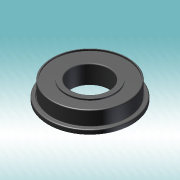
# Autodesk Inventor part: C-SFL6901ZZ
Saved by Autodesk Inventor 2015 (Build 190159000, 159)
## iProperties
Category: PARTsolutions
Company: MISUMI
Created: 2016-03-21
Part Number: C-SFL6901ZZ
Catalog Web Link: www.cadenas.de
Description: C-SFL6__ZZ, C-SFL6__AZZ, C-SFL6___ZZ-C-VALUE Stainless Steel Deep Groove Ball Bearings with Flange - Double Shielded
Vendor: MISUMI
Document SubType Name: Modeling
Designer: psAdmin
Manufacturer: MISUMI
Mass: 1.96986 g
Surface Area: 16.7276 cm^2
Volume: 1.96986 cm^3
Density: 1 g/cm^3
Material: 一般
Appearance: PSOLRGB-175-175-175
PSOL_IDENT_0: {$CADENAS_DATA\23d-libs\misumi\metric\12_bearing_holders\12_cn\c_sfl673zz.prj},195 {VTYP=3D},{NB=C-S
PSOL_IDENT_1: FL6901ZZ},{LINA=C-SFL6901ZZ},{NN=C-SFL6__ZZ, C-SFL6__AZZ, C-SFL6___ZZ},{DATE=21.07.2015 12:46:03},{G
PSOL_IDENT_2: EOMDATE=01.08.2014 01:01:00},{VERSION=},{LINEID=430},{LINESUBID=-1},{WBVAR=}  {NB=C-SFL6901ZZ},{LINA=
PSOL_IDENT_3: C-SFL6901ZZ},{KT=DUMMY},{PN=C-SFL6901ZZ},{TYPE=C-SFL6901ZZ},{BN=6901ZZ},{DD=12.0},{D=24},{B=6.0},{D1=
PSOL_IDENT_4: 26.5},{C=1.5},{RR=0.30},{B11=0.438},{D11=15.430},{D22=23.040}
NN: C-SFL6__ZZ, C-SFL6__AZZ, C-SFL6___ZZ
NT: C-VALUE Stainless Steel Deep Groove Ball Bearings with Flange - Double Shielded
NB: C-SFL6901ZZ
NBSYN: $PN.
LINA: C-SFL6901ZZ
PN: C-SFL6901ZZ
BN: 6901ZZ
DD: 12.0
D: 24
B: 6.0
D1: 26.5
C: 1.5
RR: 0.30
SUPPLIER: MISUMI
ARTICLENO: C-SFL6901ZZ
BOMINFO: C-SFL6901ZZ
CREATOR: CADENAS GmbH
Title: C-SFL6901ZZ
Author: Cadenas PARTsolutions
Comments: C-VALUE Stainless Steel Deep Groove Ball Bearings with Flange - Double Shielded
Autodesk Inventor part; units mm, degrees
ref_plane "YZ Plane" through (0, 0, 0) normal (1, 0, 0) x (0, 1, 0)
ref_plane "XZ Plane" through (0, 0, 0) normal (0, 1, 0) x (-1, 0, 0)
ref_plane "XY Plane" through (0, 0, 0) normal (0, 0, 1) x (1, 0, 0)
sketch "Sketch_1" plane through (0, 0, 0) normal (1, 0, 0) x (0, 0, -1)
  line L0 (6, 0) -> (0, 0)
  line L1 (0, 11.7) -> (0, 11.52)
  line L2 (0, 11.52) -> (0.438, 11.52)
  line L3 (0.438, 11.52) -> (0.438, 7.715)
  line L4 (0.438, 7.715) -> (0, 7.715)
  line L5 (0, 7.715) -> (0, 6.3)
  arc A0 (0, 6.3) -> (0.3, 6) centre (0.3, 6.3) ccw
  line L6 (0.3, 6) -> (5.7, 6)
  arc A1 (5.7, 6) -> (6, 6.3) centre (5.7, 6.3) ccw
  line L7 (6, 6.3) -> (6, 7.715)
  line L8 (6, 7.715) -> (5.562, 7.715)
  line L9 (5.562, 7.715) -> (5.562, 11.52)
  line L10 (5.562, 11.52) -> (6, 11.52)
  line L11 (6, 11.52) -> (6, 12.95)
  arc A2 (6, 12.95) -> (5.7, 13.25) centre (5.7, 12.95) ccw
  line L12 (5.7, 13.25) -> (4.8, 13.25)
  arc A3 (4.8, 13.25) -> (4.5, 12.95) centre (4.8, 12.95) ccw
  line L13 (4.5, 12.95) -> (4.5, 12.2)
  arc A4 (4.3, 12) -> (4.5, 12.2) centre (4.5, 12) ccw
  line L14 (4.3, 12) -> (0.3, 12)
  arc A5 (0.3, 12) -> (0, 11.7) centre (0.3, 11.7) ccw
  constraints: 30 end point, 12 point on circle, 6 centre point
revolve "Revolution1" add sketch "Sketch_1" angle 360 about axis through (0, 0, -6) along (0, 0, -1)
body "Solid1"
